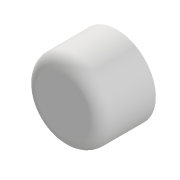
# Autodesk Inventor part: Mutter
Saved by Autodesk Inventor 2020.3 (Build 243373000, 373)
## iProperties
Created: 2021-06-01
Part Number: Mutter
Material: Generisch
Document SubType Name: Modeling
Designer: Sven
Density: 1 g/cm^3
Appearance: Vorgabe
Author: Sven
Autodesk Inventor part; units mm, degrees
ref_plane "YZ Plane" through (0, 0, 0) normal (1, 0, 0) x (0, 1, 0)
ref_plane "XZ Plane" through (0, 0, 0) normal (0, 1, 0) x (-1, 0, 0)
ref_plane "XY Plane" through (0, 0, 0) normal (0, 0, 1) x (1, 0, 0)
sketch "Skizze1" plane through (0, 0, 0) normal (0, 0, 1) x (1, 0, 0)
  circle A0 centre (0, -2.5) radius 5 projected
  circle A1 centre (0, -2.5) radius 2.5 projected
  circle A2 centre (0, -2.5) radius 6.5
  point P0 (0, 0)
  dimension "d0" = 13
  constraints: 1 centre point, 1 coincident, 1 vertical alignment
  measures "d0" diameter of A2
extrude "Extrusion1" add sketch "Skizze1" against normal blind 7 contours A2
thread "Gewinde1" size "M10x1.5" class "6H" standard "ANSI Metric M Profile" full length
sketch "Skizze2" plane through (0, -2.5, 0) normal (0, 0, 1) x (1, 0, 0)
  circle A0 centre (0, 0) radius 6.5
  point P0 (0, 2.5)
  constraints: 1 centre point
extrude "Extrusion2" add sketch "Skizze2" along normal blind 2
fillet "Rundung1" radius 2 1 edges at (-6.5, -2.5, 2)
